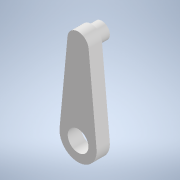
# Autodesk Inventor part: shatun_lidar
Saved by Autodesk Inventor 2022 (Build 260153000, 153)
## iProperties
Created: 2024-10-20
Part Number: shatun_lidar
Material: Типовые
Document SubType Name: Modeling
Designer: Andrey
Density: 1 g/cm^3
Appearance: По умолчанию
Author: Andrey
Autodesk Inventor part; units mm, degrees
ref_plane "YZ Plane" through (0, 0, 0) normal (1, 0, 0) x (0, 1, 0)
ref_plane "XZ Plane" through (0, 0, 0) normal (0, 1, 0) x (-1, 0, 0)
ref_plane "XY Plane" through (0, 0, 0) normal (0, 0, 1) x (1, 0, 0)
sketch "Эскиз1" plane through (0, 0, 0) normal (0, 0, 1) x (1, 0, 0)
  circle A0 centre (0, 0) radius 4 projected
  arc A1 (-13.2, 4.5) -> (-13.2, -4.5) centre (-13.2, 0) ccw projected
  line L0 (-13.2, -4.5) -> (1.3, -4.5) projected
  arc A2 (1.3, -4.5) -> (1.3, 4.5) centre (1.3, 0) ccw projected
  line L1 (1.3, 4.5) -> (-13.2, 4.5) projected
  circle A3 centre (0, 6.5601) radius 1.1 projected
  arc A4 (-8.1687, 23.1585) -> (8.1687, 23.1585) centre (0, 35.5) ccw projected
  arc A5 (10.1004, 20.2399) -> (8.1687, 23.1585) centre (9.1346, 21.6992) ccw projected
  arc A6 (-10.1004, 20.2399) -> (10.1004, 20.2399) centre (0, 35.5) ccw projected
  arc A7 (-8.1687, 23.1585) -> (-10.1004, 20.2399) centre (-9.1346, 21.6992) ccw projected
  line L2 (13.75, 27.1) -> (13.75, 10.8) projected
  line L3 (13.75, 27.1) -> (-13.75, 27.1) projected
  line L4 (-13.75, 27.1) -> (-13.75, 10.8) projected
  line L5 (-13.75, 10.8) -> (-0.7414, 4.9199) projected
  arc A8 (-0.7414, 4.9199) -> (0.7414, 4.9199) centre (0, 6.5601) ccw projected
  line L6 (0.7414, 4.9199) -> (13.75, 10.8) projected
  circle A9 centre (0, 0) radius 14.9209
  circle A10 centre (-9.898, 8.3054) radius 2
  circle A11 centre (0, 0) radius 1.5
  circle A12 centre (0, 0) radius 3.5
  line L7 (-86.0992, 75.6487) -> (86.0992, -4.6487) projected
  line L8 (-1.991, 16.0319) -> (-3.4843, 0.3314)
  line L9 (3.4843, 0.3314) -> (1.991, 16.0319)
  circle A13 centre (0, 6.5601) radius 1.25
  line L10 (1.25, 15.8425) -> (1.25, 6.5601)
  line L11 (-1.25, 6.5601) -> (-1.25, 15.8425)
  arc A14 (14.6884, 10.9864) -> (-14.6884, 10.9864) centre (0, 0) ccw projected
  arc A15 (14.8244, 8.1933) -> (14.6884, 10.9864) centre (12.6864, 9.489) ccw projected
  arc A16 (-14.6884, 10.9864) -> (-15.006, 8.5565) centre (-12.6864, 9.489) ccw projected
  circle A17 centre (0, 0) radius 15.8425
  circle A18 centre (0, 15.8425) radius 1.25
  circle A19 centre (0, 15.8425) radius 2
  line L12 (0, 7.2054) -> (0, 9.4054) projected
  line L13 (0, -12.9209) -> (0, 12.9209) projected
  point P0 (0, 0)
  point P1 (86.0992, -4.6487)
  point P2 (-1.25, 15.7932)
  point P3 (-1.249, 15.7932)
  point P4 (1.249, 15.7932)
  point P5 (1.25, 15.7932)
  point P6 (2.0213, 15.7131)
  point P7 (1.996, 15.7163)
  point P8 (-1.996, 15.7163)
  point P9 (-2.0213, 15.7131)
  dimension "d0" = 4
  dimension "d1" = 3
  dimension "d2" = 7
  dimension "d6" = 2.5
  dimension "d7" = 2.5
  dimension "d8" = 4
  constraints: 10 point on circle, 9 tangent, 8 centre point, 8 end point, 5 coincident, 2 other
  measures "d0" diameter of A10
  measures "d1" diameter of A11
  measures "d2" diameter of A12
  measures "d6" diameter of A13
  measures "d7" diameter of A18
  measures "d8" diameter of A19
extrude "Выдавливание1" add sketch "Эскиз1" along normal blind 2.5 contours L9 A12 L13 A0 | A0 L13 L1 A2 L9 | L13 A12 L8 A0 | A0 L8 L1 L13 | A12 L13 A11 | A2 L1 L13 A8 L6 L9 | A12 L13 A11 | L1 L8 L5 A8 L13 | L6 A8 L13 A13 L10 A19 A9 L9 | A8 L5 L8 A9 A19 L11 A13 L13 | A9 A19 A17 L9 | L13 A3 L12 A13 | A13 L12 A3 L13 | A19 L10 A9 | A9 L10 A17 A19 | A17 A19 L9 | L8 A17 A19 A9 | L11 A19 L10 A13 | L13 L12 A3 | A3 L12 L13 | L10 A19 L11 A9 A18 | A9 A18 L10 | A17 L10 A18 L11 A19 A6 | A19 A17 L11 A9 | A9 L11 A19 | L8 A19 A17 | A18 A9 | A9 A18 A17 | A17 L11 A18 L10 | A6 A19 | L11 A18 A9 picked at (0.3204, 3.7943) picked at (-0.3204, 3.7943)
sketch "Эскиз2" plane through (0, 0, 0) normal (0, 0, -1) x (-1, 0, 0)
  circle A0 centre (0, 0) radius 14.9209
  arc A1 (1.991, 16.0319) -> (-1.991, 16.0319) centre (0, 12.9209) ccw projected
  circle A2 centre (0, 0) radius 1.95
  arc A3 (-3.4843, 0.3314) -> (3.4843, 0.3314) centre (0, 0) ccw projected
  line L0 (1.991, 16.0319) -> (3.4843, 0.3314) projected
  arc A4 (1.991, 16.0319) -> (-1.991, 16.0319) centre (0, 15.8425) ccw projected
  line L1 (-3.4843, 0.3314) -> (-1.991, 16.0319) projected
  point P0 (0, 0)
  dimension "d9" = 3.9
  constraints: 2 centre point, 2 other
  measures "d9" diameter of A2
extrude "Выдавливание2" cut sketch "Эскиз2" against normal blind 3 contours A2
sketch "Эскиз3" plane through (0, 0, 0) normal (0, 0, -1) x (-1, 0, 0)
  circle A0 centre (0, 0) radius 1.95 projected
  arc A1 (-3.4843, 0.3314) -> (3.4843, 0.3314) centre (0, 0) ccw projected
  line L0 (1.991, 16.0319) -> (3.4843, 0.3314) projected
  arc A2 (1.991, 16.0319) -> (-1.991, 16.0319) centre (0, 15.8425) ccw projected
  line L1 (-3.4843, 0.3314) -> (-1.991, 16.0319) projected
  circle A3 centre (0, 15.8425) radius 1.5
  point P0 (0, 0)
  dimension "d12" = 3
  constraints: 1 centre point, 1 coincident
  measures "d12" diameter of A3
extrude "Выдавливание3" add sketch "Эскиз3" along normal blind 2 contours A3
